Hanger Test (Autodesk Fusion 360 design; units mm, degrees)
Autodesk Fusion 360 part; units mm, degrees
note: some values were not read from the file. Set by a fixed rule: which sketch regions a step uses.
sketch "Sketch1" plane through (0, 0, 0) normal (0, 0, 1) x (1, 0, 0)
  line L0 (0, 0) -> (50, 0)
  line L1 (50, 0) -> (50, 25)
  line L2 (50, 25) -> (0, 25)
  line L3 (0, 25) -> (0, 0)
  circle A0 centre (12, 10) radius 2.5
  circle A1 centre (38, 10) radius 2.5
  line L4 (0, 25) -> (50, 25)
  line L5 (50, 25) -> (50, 18)
  line L6 (50, 18) -> (0, 18)
  line L7 (0, 18) -> (0, 25)
  circle A2 centre (6.25, 18) radius 3
  circle A3 centre (13.75, 18) radius 3
  circle A4 centre (21.25, 18) radius 3
  circle A5 centre (28.75, 18) radius 3
  circle A6 centre (36.25, 18) radius 3
  circle A7 centre (43.75, 18) radius 3
  dimension "d1" = 50
  dimension "d2" = 25
  dimension "d3" = 5
  dimension "d4" = 12
  dimension "d5" = 5
  dimension "d6" = 12
  dimension "d7" = 7
  dimension "d8" = 6
  dimension "d9" = 6
  dimension "d10" = 7.5
  dimension "d11" = 6
  dimension "d12" = 6
  dimension "d13" = 6
  dimension "d14" = 6
  dimension "d15" = 7.5
  dimension "d16" = 7.5
  dimension "d17" = 7.5
  dimension "d18" = 7.5
  dimension "d19" = 6.25
  dimension "d20" = 10
  dimension "d21" = 10
  constraint horizontal L0
  constraint vertical L1
  constraint horizontal L2
  constraint vertical L3
  constraint coincident L0.start L3.end
  constraint horizontal L4
  constraint vertical L5
  constraint horizontal L6
  constraint vertical L7
  constraint coincident L6 A2.centre
  constraint coincident L6 A3.centre
  constraint coincident L6 A4.centre
  constraint coincident L6 A5.centre
  constraint coincident L6 A6.centre
  constraint coincident L6 A7.centre
  measures "d1" distance of L0.start L0.end
  measures "d2" distance of L0.start L2.end
  measures "d3" diameter of A0
  measures "d4" distance of L3 A0.centre
  measures "d5" diameter of A1
  measures "d6" distance of L1 A1.centre
  measures "d7" distance of L2.end L6.end
  measures "d8" diameter of A2
  measures "d9" diameter of A3
  measures "d10" distance of A2.centre A3.centre
  measures "d11" diameter of A4
  measures "d12" diameter of A5
  measures "d13" diameter of A6
  measures "d14" diameter of A7
  measures "d15" distance of A3.centre A4.centre
  measures "d16" distance of A4.centre A5.centre
  measures "d17" distance of A5.centre A6.centre
  measures "d18" distance of A6.centre A7.centre
  measures "d19" distance of L3 A2.centre
  measures "d20" distance of L0 A0.centre
  measures "d21" distance of L0 A1.centre
extrude "Extrude1" add sketch "Sketch1" along normal blind 2
extrude "Extrude2" add sketch "Sketch1" along normal blind 12 contours L1 L2 L3 L4 L5 L6 L7 A2 A3 A4 A5 A6 A7
